Autodesk Inventor part; units mm, degrees
(part 2 of 2)
sketch "Sketch5" plane through (0, 0, 4) normal (0, 0, 1) x (1, 0, 0)
  line L0 (-45.7847, 120.7797) -> (-46.0213, 121.5085) projected
  line L1 (-46.0213, 121.5085) -> (-48.3698, 120.7462) projected
  line L2 (-48.3698, 120.7462) -> (-48.6483, 121.6043) projected
  line L3 (-48.6483, 121.6043) -> (-49.2008, 121.4249) projected
  line L4 (-49.2008, 121.4249) -> (-48.4072, 118.98) projected
  line L5 (-48.4072, 118.98) -> (-47.8547, 119.1593) projected
  line L6 (-47.8547, 119.1593) -> (-48.1332, 120.0174) projected
  line L7 (-48.1332, 120.0174) -> (-45.7847, 120.7797) projected
  line L8 (-64.9446, 81.0789) -> (-65.476, 81.0789) projected
  line L9 (-65.476, 81.0789) -> (-65.476, 80.4511) projected
  line L10 (-65.476, 80.4511) -> (-68.002, 80.4511) projected
  line L11 (-68.002, 80.4511) -> (-68.002, 79.7837) projected
  line L12 (-67.5868, 79.0645) -> (-67.09, 79.0645) projected
  line L13 (-67.09, 79.0645) -> (-67.09, 79.7071) projected
  line L14 (-67.09, 79.7071) -> (-65.476, 79.7071) projected
  line L15 (-65.476, 79.7071) -> (-65.476, 79.0645) projected
  line L16 (-65.476, 79.0645) -> (-64.9446, 79.0645) projected
  line L17 (-64.9446, 79.0645) -> (-64.9446, 81.0789) projected
  line L18 (-68.6353, 113.1682) -> (-73.2476, 116.7073) projected
  arc A0 (-73.2476, 116.7073) -> (-70.5597, 118.9777) centre (-77.1049, 124) ccw projected
  line L19 (-70.5597, 118.9777) -> (-66.1963, 115.6295) projected
  arc A1 (-68.6353, 113.1682) -> (-66.1963, 115.6295) centre (-77.1049, 124) ccw projected
  arc A2 (-69.0623, 122.1616) -> (-69.3017, 126.6781) centre (-77.1049, 124) ccw projected
  line L20 (-69.3017, 126.6781) -> (-63.4725, 122.2053) projected
  arc A3 (-64.4501, 118.6225) -> (-63.4725, 122.2053) centre (-77.1049, 124) ccw projected
  line L21 (-64.4501, 118.6225) -> (-69.0623, 122.1616) projected
  arc A4 (-63.6117, 126.6449) -> (-78.0424, 137.718) centre (-77.1049, 124) ccw projected
  line L22 (-63.6117, 126.6449) -> (-78.0424, 137.718) projected
  arc A5 (-76.5376, 132.2305) -> (-80.9622, 131.2927) centre (-77.1049, 124) ccw projected
  line L23 (-80.9622, 131.2927) -> (-85.5745, 134.8318) projected
  arc A6 (-82.3668, 136.7033) -> (-85.5745, 134.8318) centre (-77.1049, 124) ccw projected
  line L24 (-82.3668, 136.7033) -> (-76.5376, 132.2305) projected
  arc A7 (-83.6501, 129.0223) -> (-77.6721, 115.7695) centre (-77.1049, 124) ccw projected
  line L25 (-77.6721, 115.7695) -> (-71.843, 111.2967) projected
  arc A8 (-76.1674, 110.282) -> (-71.843, 111.2967) centre (-77.1049, 124) ccw projected
  line L26 (-76.1674, 110.282) -> (-85.575, 117.5007) projected
  line L27 (-85.575, 117.5007) -> (-88.0135, 115.6295) projected
  arc A9 (-88.0135, 132.3705) -> (-88.0135, 115.6295) centre (-77.1049, 124) ccw projected
  line L28 (-88.0135, 132.3705) -> (-83.6501, 129.0223) projected
  circle A10 centre (-77.1049, 124) radius 15.25 projected
  line L29 (-4.0321, 74.7867) -> (-4.0249, 74.7738) projected
  line L30 (-4.0249, 74.7738) -> (-5.6933, 73.843) projected
  line L31 (-5.6933, 73.843) -> (-5.7006, 73.8559) projected
  line L32 (-6.2765, 73.7214) -> (-5.8165, 72.8969) projected
  line L33 (-5.8165, 72.8969) -> (-3.153, 74.3828) projected
  line L34 (-3.153, 74.3828) -> (-3.6178, 75.216) projected
  line L35 (-5.3035, 85.1893) -> (-5.412, 84.998) projected
  line L36 (-5.412, 84.998) -> (-6.1259, 85.4027) projected
  line L37 (-6.1259, 85.4027) -> (-5.9991, 85.6263) projected
  line L38 (-2.9465, 85.964) -> (-4.5812, 85.7117) projected
  line L39 (-6.3848, 86.0836) -> (-6.9894, 85.0172) projected
  line L40 (-6.9894, 85.0172) -> (-4.3362, 83.5129) projected
  line L41 (-4.3362, 83.5129) -> (-3.9607, 84.1751) projected
  line L42 (-3.9607, 84.1751) -> (-4.9347, 84.7273) projected
  line L43 (-4.9347, 84.7273) -> (-4.7982, 84.9682) projected
  line L44 (-4.7982, 84.9682) -> (-3.4061, 85.1534) projected
  line L45 (-3.4061, 85.1534) -> (-2.9465, 85.964) projected
  line L46 (-47.1878, 118.4663) -> (-47.2251, 118.5216) projected
  line L47 (-47.2251, 118.5216) -> (-47.8025, 118.1312) projected
  line L48 (-44.8979, 117.3921) -> (-44.8591, 117.3348) projected
  line L49 (-44.8591, 117.3348) -> (-44.2572, 117.7418) projected
  line L50 (-47.5223, 123.4503) -> (-48.537, 123.7435) projected
  line L51 (-48.537, 123.7435) -> (-47.5351, 124.0755) projected
  line L52 (-47.5351, 124.0755) -> (-47.5223, 123.4503) projected
  line L53 (-46.323, 122.3501) -> (-46.3387, 123.1161) projected
  line L54 (-46.3387, 123.1161) -> (-46.9654, 123.2961) projected
  line L55 (-46.9654, 123.2961) -> (-46.985, 124.2549) projected
  line L56 (-46.985, 124.2549) -> (-46.3662, 124.4579) projected
  line L57 (-46.3662, 124.4579) -> (-46.3824, 125.2462) projected
  line L58 (-46.3824, 125.2462) -> (-49.4106, 124.1533) projected
  line L59 (-49.4106, 124.1533) -> (-49.3935, 123.318) projected
  line L60 (-49.3935, 123.318) -> (-46.323, 122.3501) projected
  line L61 (-47.6082, 126.9904) -> (-47.6727, 126.7801) projected
  line L62 (-47.6727, 126.7801) -> (-48.4572, 127.021) projected
  line L63 (-48.4572, 127.021) -> (-48.3817, 127.2667) projected
  line L64 (-45.4742, 128.2561) -> (-47.0157, 127.6565) projected
  line L65 (-48.8571, 127.6299) -> (-49.217, 126.458) projected
  line L66 (-49.217, 126.458) -> (-46.3014, 125.5626) projected
  line L67 (-46.3014, 125.5626) -> (-46.0779, 126.2903) projected
  line L68 (-46.0779, 126.2903) -> (-47.1482, 126.619) projected
  line L69 (-47.1482, 126.619) -> (-47.0669, 126.8836) projected
  line L70 (-47.0669, 126.8836) -> (-45.7477, 127.3653) projected
  line L71 (-45.7477, 127.3653) -> (-45.4742, 128.2561) projected
  line L72 (-44.9597, 128.9002) -> (-44.5276, 129.5329) projected
  line L73 (-44.5276, 129.5329) -> (-46.5666, 130.9254) projected
  line L74 (-46.5666, 130.9254) -> (-46.0578, 131.6704) projected
  line L75 (-46.0578, 131.6704) -> (-46.5375, 131.998) projected
  line L76 (-46.5375, 131.998) -> (-47.9871, 129.8752) projected
  line L77 (-47.9871, 129.8752) -> (-47.5075, 129.5477) projected
  line L78 (-47.5075, 129.5477) -> (-46.9987, 130.2927) projected
  line L79 (-46.9987, 130.2927) -> (-44.9597, 128.9002) projected
  circle A11 centre (-37.1049, 124) radius 6.25 projected
  circle A12 centre (4.3054, 80) radius 6.25 projected
  circle A13 centre (-57.1049, 124) radius 2.5 projected
  circle A14 centre (-55.6946, 80) radius 6.25 projected
  circle A15 centre (-25.6946, 80) radius 6.25 projected
  line L80 (-62.1049, 160) -> (-62.1049, 156) projected
  line L81 (-62.1049, 156) -> (-48.2523, 156) projected
  line L82 (-48.2523, 156) -> (-48.2523, 151.2) projected
  line L83 (-48.2523, 151.2) -> (-49.4523, 151.2) projected
  line L84 (-49.4523, 151.2) -> (-49.4523, 148.8) projected
  line L85 (-49.4523, 148.8) -> (-48.2523, 148.8) projected
  line L86 (-48.2523, 148.8) -> (-48.2523, 144) projected
  line L87 (-48.2523, 144) -> (-45.2523, 144) projected
  line L88 (-45.2523, 144) -> (-45.2523, 148.8) projected
  line L89 (-45.2523, 148.8) -> (-44.0523, 148.8) projected
  line L90 (-44.0523, 148.8) -> (-44.0523, 151.2) projected
  line L91 (-44.0523, 151.2) -> (-45.2523, 151.2) projected
  line L92 (-45.2523, 151.2) -> (-45.2523, 156) projected
  line L93 (-45.2523, 156) -> (-17.5472, 156) projected
  line L94 (-17.5472, 156) -> (-17.5472, 151.2) projected
  line L95 (-17.5472, 151.2) -> (-18.7472, 151.2) projected
  line L96 (-18.7472, 151.2) -> (-18.7472, 148.8) projected
  line L97 (-18.7472, 148.8) -> (-17.5472, 148.8) projected
  line L98 (-17.5472, 148.8) -> (-17.5472, 144) projected
  line L99 (-17.5472, 144) -> (-14.5472, 144) projected
  line L100 (-14.5472, 144) -> (-14.5472, 148.8) projected
  line L101 (-14.5472, 148.8) -> (-13.3472, 148.8) projected
  line L102 (-13.3472, 148.8) -> (-13.3472, 151.2) projected
  line L103 (-13.3472, 151.2) -> (-14.5472, 151.2) projected
  line L104 (-14.5472, 151.2) -> (-14.5472, 156) projected
  line L105 (-14.5472, 156) -> (-0.6946, 156) projected
  line L106 (-0.6946, 156) -> (-0.6946, 160) projected
  line L107 (-0.6946, 160) -> (39.3054, 160) projected
  line L108 (39.3054, 160) -> (39.3054, 0) projected
  line L109 (39.3054, 0) -> (-0.6946, 0) projected
  line L110 (-0.6946, 0) -> (-0.6946, 4) projected
  line L111 (-0.6946, 4) -> (-14.5472, 4) projected
  line L112 (-14.5472, 4) -> (-14.5472, 8.8) projected
  line L113 (-14.5472, 8.8) -> (-13.3472, 8.8) projected
  line L114 (-13.3472, 8.8) -> (-13.3472, 11.2) projected
  line L115 (-13.3472, 11.2) -> (-14.5472, 11.2) projected
  line L116 (-14.5472, 11.2) -> (-14.5472, 16) projected
  line L117 (-14.5472, 16) -> (-17.5472, 16) projected
  line L118 (-17.5472, 16) -> (-17.5472, 11.2) projected
  line L119 (-17.5472, 11.2) -> (-18.7472, 11.2) projected
  line L120 (-18.7472, 11.2) -> (-18.7472, 8.8) projected
  line L121 (-18.7472, 8.8) -> (-17.5472, 8.8) projected
  line L122 (-17.5472, 8.8) -> (-17.5472, 4) projected
  line L123 (-17.5472, 4) -> (-45.2523, 4) projected
  line L124 (-45.2523, 4) -> (-45.2523, 8.8) projected
  line L125 (-45.2523, 8.8) -> (-44.0523, 8.8) projected
  line L126 (-44.0523, 8.8) -> (-44.0523, 11.2) projected
  line L127 (-44.0523, 11.2) -> (-45.2523, 11.2) projected
  line L128 (-45.2523, 11.2) -> (-45.2523, 16) projected
  line L129 (-45.2523, 16) -> (-48.2523, 16) projected
  line L130 (-48.2523, 16) -> (-48.2523, 11.2) projected
  line L131 (-48.2523, 11.2) -> (-49.4523, 11.2) projected
  line L132 (-49.4523, 11.2) -> (-49.4523, 8.8) projected
  line L133 (-49.4523, 8.8) -> (-48.2523, 8.8) projected
  line L134 (-48.2523, 8.8) -> (-48.2523, 4) projected
  line L135 (-48.2523, 4) -> (-62.1049, 4) projected
  line L136 (-62.1049, 4) -> (-62.1049, 0) projected
  line L137 (-62.1049, 0) -> (-102.1049, 0) projected
  line L138 (-102.1049, 0) -> (-102.1049, 160) projected
  line L139 (-102.1049, 160) -> (-62.1049, 160) projected
  line L140 (-86.2764, 122.7383) -> (-88.7065, 122.3008) projected
  line L141 (-88.7065, 122.3008) -> (-88.8664, 123.1887) projected
  line L142 (-88.8664, 123.1887) -> (-89.438, 123.0858) projected
  line L143 (-89.438, 123.0858) -> (-88.9826, 120.5559) projected
  line L144 (-88.9826, 120.5559) -> (-88.411, 120.6588) projected
  line L145 (-88.411, 120.6588) -> (-88.5708, 121.5467) projected
  line L146 (-88.5708, 121.5467) -> (-86.1407, 121.9842) projected
  line L147 (-86.1407, 121.9842) -> (-86.2764, 122.7383) projected
  line L148 (-87.8439, 119.882) -> (-87.8735, 119.9418) projected
  line L149 (-87.8735, 119.9418) -> (-88.4984, 119.6331) projected
  line L150 (-85.7206, 118.5077) -> (-85.6899, 118.4456) projected
  line L151 (-85.6899, 118.4456) -> (-85.0384, 118.7675) projected
  line L152 (-88.6263, 128.4355) -> (-85.8847, 127.099) projected
  line L153 (-85.8847, 127.099) -> (-85.549, 127.7878) projected
  line L154 (-85.549, 127.7878) -> (-86.4465, 128.2253) projected
  line L155 (-86.4465, 128.2253) -> (-86.2711, 128.5852) projected
  line L156 (-88.1075, 129.4997) -> (-88.6263, 128.4355) projected
  line L157 (-86.9337, 128.5233) -> (-86.9575, 128.4744) projected
  line L158 (-86.9575, 128.4744) -> (-87.7796, 128.8751) projected
  line L159 (-87.7796, 128.8751) -> (-87.7319, 128.9729) projected
  point P0 (0, 0)
  constraints: 114 other
body "Solid1"
